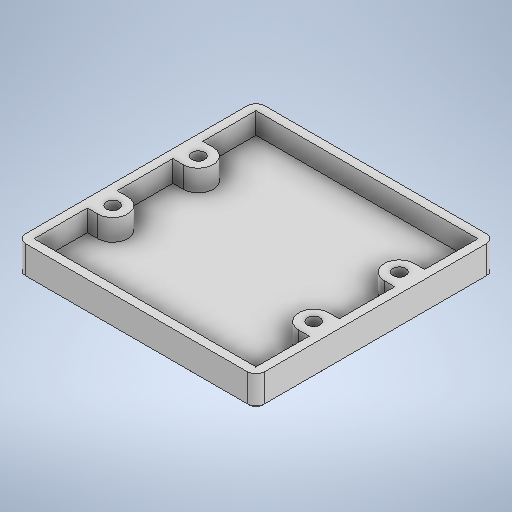
# Autodesk Inventor part: BlindCover
Saved by Autodesk Inventor 2025.2 (Build 292293000, 293)
## iProperties
Created: 2025-05-07
Part Number: BlindCover
Material: Generisch
Document SubType Name: Modeling
Designer: Jannis
Density: 1 g/cm^3
Appearance: Vorgabe
Author: Jannis
Autodesk Inventor part; units mm, degrees
ref_plane "YZ Plane" through (0, 0, 0) normal (1, 0, 0) x (0, 1, 0)
ref_plane "XZ Plane" through (0, 0, 0) normal (0, 1, 0) x (-1, 0, 0)
ref_plane "XY Plane" through (0, 0, 0) normal (0, 0, 1) x (1, 0, 0)
sketch "Skizze1" plane through (0, 0, 0) normal (0, 0, 1) x (1, 0, 0)
  line L0 (-27.95, 27.95) -> (27.95, 27.95)
  line L1 (27.95, 27.95) -> (27.95, -27.95)
  line L2 (27.95, -27.95) -> (-27.95, -27.95)
  line L3 (-27.95, -27.95) -> (-27.95, 27.95)
  line L4 (-27.95, 27.95) -> (27.95, -27.95) construction
  line L5 (27.95, 27.95) -> (-27.95, -27.95) construction
  point P0 (0, 0)
  dimension "d0" = 55.9
  dimension "d1" = 55.9
  constraints: 12 end point, 2 midpoint, 2 parallel, 1 horizontal, 1 perpendicular
  measures "d0" distance of L0.start L0.end
  measures "d1" distance of L0.end L1.end
extrude "Extrusion1" add sketch "Skizze1" along normal blind 2
sketch "Skizze2" plane through (0, 0, 2) normal (0, 0, 1) x (1, 0, 0)
  line L0 (-27.95, -27.95) -> (27.95, -27.95) projected
  line L1 (27.95, -27.95) -> (27.95, 27.95) projected
  line L2 (27.95, 27.95) -> (-27.95, 27.95) projected
  line L3 (-27.95, 27.95) -> (-27.95, -27.95) projected
  line L4 (-25.95, 25.95) -> (25.95, 25.95)
  line L5 (25.95, 25.95) -> (25.95, -25.95)
  line L6 (25.95, -25.95) -> (-25.95, -25.95)
  line L7 (-25.95, -25.95) -> (-25.95, 25.95)
  point P0 (0, 0)
  dimension "d4" = 2
  constraints: 8 end point, 3 other
  measures "d4" distance between parallel lines of L2 L4
extrude "Extrusion2" add sketch "Skizze2" along normal blind 5
fillet "Rundung1" radius 2 4 edges at (-27.95, -27.95, 3.5) (27.95, -27.95, 3.5) (27.95, 27.95, 3.5) (-27.95, 27.95, 3.5)
sketch "Skizze5" plane through (0, 0, 2) normal (0, 0, 1) x (1, 0, 0)
  line L0 (-23.5, 10) -> (23.5, 10) construction
  line L1 (23.5, 10) -> (23.5, -10) construction
  line L2 (23.5, -10) -> (-23.5, -10) construction
  line L3 (-23.5, -10) -> (-23.5, 10) construction
  line L4 (-23.5, 10) -> (23.5, -10) construction
  line L5 (23.5, 10) -> (-23.5, -10) construction
  arc A0 (-23.5, -13.5) -> (-23.5, -6.5) centre (-23.5, -10) ccw
  arc A1 (-23.5, 6.5) -> (-23.5, 13.5) centre (-23.5, 10) ccw
  arc A2 (23.5, 13.5) -> (23.5, 6.5) centre (23.5, 10) ccw
  arc A3 (23.5, -6.5) -> (23.5, -13.5) centre (23.5, -10) ccw
  line L6 (-25.95, 25.95) -> (25.95, 25.95) projected
  line L7 (-25.95, -25.95) -> (-25.95, 25.95) projected
  line L8 (25.95, -25.95) -> (-25.95, -25.95) projected
  line L9 (25.95, 25.95) -> (25.95, -25.95) projected
  line L10 (23.5, -13.5) -> (25.95, -13.5)
  line L11 (23.5, -6.5) -> (25.95, -6.5)
  line L12 (23.5, 6.5) -> (25.95, 6.5)
  line L13 (23.5, 13.5) -> (25.95, 13.5)
  line L14 (-23.5, 13.5) -> (-25.95, 13.5)
  line L15 (-23.5, 6.5) -> (-25.95, 6.5)
  line L16 (-23.5, -6.5) -> (-25.95, -6.5)
  line L17 (-23.5, -13.5) -> (-25.95, -13.5)
  point P0 (0, 0)
  point P1 (-23.95, 25.95)
  point P2 (23.95, 25.95)
  point P3 (-25.95, -23.95)
  point P4 (-25.95, 23.95)
  point P5 (23.95, -25.95)
  point P6 (-23.95, -25.95)
  point P7 (25.95, 23.95)
  point P8 (25.95, -23.95)
  dimension "d17" = 47
  dimension "d18" = 20
  dimension "d19" = 7
  dimension "d20" = 7
  dimension "d21" = 7
  dimension "d22" = 7
  constraints: 28 end point, 12 point on line, 8 point on circle, 7 tangent, 5 perpendicular, 4 centre point, 4 coincident, 4 horizontal, 2 midpoint, 2 parallel
  measures "d17" distance of L0.start L0.end
  measures "d18" distance of L0.end L1.end
  measures "d19" diameter of A0
  measures "d20" diameter of A1
  measures "d21" diameter of A2
  measures "d22" diameter of A3
extrude "Extrusion3" add sketch "Skizze5" along normal blind 5 contours L17 L7 L16 A0 | L7 L14 A1 L15 | L10 A3 L11 L9 | L12 A2 L13 L9
sketch "Skizze3" plane through (0, 0, 0) normal (0, 0, -1) x (-1, 0, 0)
  line L0 (23.5, 10) -> (-23.5, 10)
  line L1 (-23.5, 10) -> (-23.5, -10)
  line L2 (-23.5, -10) -> (23.5, -10)
  line L3 (23.5, -10) -> (23.5, 10)
  line L4 (23.5, 10) -> (-23.5, -10) construction
  line L5 (-23.5, 10) -> (23.5, -10) construction
  point P0 (0, 0)
  dimension "d8" = 47
  dimension "d9" = 20
  constraints: 12 end point, 2 midpoint, 2 parallel, 1 horizontal, 1 perpendicular
  measures "d8" distance of L0.start L0.end
  measures "d9" distance of L1.end L0.end
hole "Bohrung1" at (23.5, -10, 0) at (23.5, 10, 0) at (-23.5, 10, 0) at (-23.5, -10, 0) direction (0, 0, 1) diameter 3 end through all counterbore diameter 6 counterbore depth 2
chamfer "Fasen1" distance 0.5 angle 45 12 edges at (0, -27.95, 0) (27.3642, -27.3642, 0) (27.95, 0, 0) (27.3642, 27.3642, 0) (0, 27.95, 0) (-27.3642, 27.3642, 0) (-27.95, 0, 0) (-27.3642, -27.3642, 0) (-23.5, -13, 0) (23.5, -13, 0) (-23.5, 7, 0) (23.5, 7, 0)
